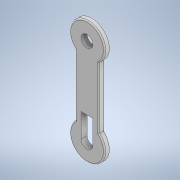
# Autodesk Inventor part: First arm
Saved by Autodesk Inventor 2022 (Build 260153000, 153)
## iProperties
Created: 2022-01-28
Part Number: First arm
Material: Generic
Document SubType Name: Modeling
Designer: Alexa
Density: 1 g/cm^3
Appearance: Default
Author: Alexa
Autodesk Inventor part; units mm, degrees
ref_plane "YZ Plane" through (0, 0, 0) normal (1, 0, 0) x (0, 1, 0)
ref_plane "XZ Plane" through (0, 0, 0) normal (0, 1, 0) x (-1, 0, 0)
ref_plane "XY Plane" through (0, 0, 0) normal (0, 0, 1) x (1, 0, 0)
sketch "Sketch1" plane through (0, 0, 0) normal (0, 0, 1) x (1, 0, 0)
  line L0 (0, 0) -> (20, 0)
  line L1 (20, 0) -> (20, 41)
  line L2 (20, 41) -> (0, 41)
  line L3 (0, 41) -> (0, 0)
  circle A0 centre (10, 0) radius 30
  circle A1 centre (10, 0) radius 10
  line L4 (10, 0) -> (30, 0)
  line L5 (30, 0) -> (30, 150)
  line L6 (30, 150) -> (10, 150)
  line L7 (10, 150) -> (10, 0)
  line L8 (10, 0) -> (-10, 0)
  line L9 (-10, 0) -> (-10, 150)
  line L10 (-10, 150) -> (10, 150)
  line L11 (10, 150) -> (10, 0)
  circle A2 centre (10, 150) radius 30
  circle A3 centre (10, 150) radius 10
  point P0 (30, 22.3607)
  point P1 (30, 127.6393)
  point P2 (-10, 127.6393)
  point P3 (-10, 22.3607)
  dimension "d0" = 20
  dimension "d1" = 41
  dimension "d2" = 60
  dimension "d3" = 20
  dimension "d4" = 150
  dimension "d5" = 20
  dimension "d6" = 150
  dimension "d7" = 60
  dimension "d8" = 20
  constraints: 24 end point, 6 parallel, 3 centre point, 3 coincident, 3 horizontal, 3 perpendicular, 1 horizontal alignment, 1 midpoint, 2 other
  measures "d0" distance of L2.end L1.end
  measures "d1" distance of L1.end L0.end
  measures "d2" diameter of A0
  measures "d3" distance of L6.end L5.end
  measures "d4" distance of L5.end L4.end
  measures "d5" distance of L9.end L10.end
  measures "d6" distance of L8.end L9.end
  measures "d7" diameter of A2
  measures "d8" diameter of A3
extrude "Extrusion1" add sketch "Sketch1" along normal blind 10 contours L8 L9 A0 L3 | L3 A0 L7 A1 | A1 L4 L5 A0 L9 L8 | A0 L9 A2 L7 L2 L3 | L3 L2 L7 A0 | A1 L7 A0 L1 | L1 A0 L5 L4 | L7 L2 L1 A0 | L1 L2 L7 A2 L5 A0 | A2 L5 L6 A3 L10 L9 | L9 L10 A3 L7 A2 | L7 A3 L6 L5 A2
fillet "Fillet1" radius 2 8 edges at (10, 180, 10) (-10, 75, 10) (10, -30, 10) (10, -30, 0) (-10, 75, 0) (10, 180, 0) (30, 75, 0) (30, 75, 10)
sketch "Sketch2" plane through (0, 0, 10) normal (0, 0, 1) x (1, 0, 0)
  line L0 (0, 0) -> (20, 0)
  line L1 (20, 0) -> (20, 40.5)
  line L2 (20, 40.5) -> (0, 40.5)
  line L3 (0, 40.5) -> (0, 0)
  dimension "d12" = 20
  dimension "d13" = 40.5
  constraints: 8 end point, 2 parallel, 1 horizontal, 1 perpendicular
  measures "d12" distance of L2.end L1.end
  measures "d13" distance of L1.end L0.end
extrude "Extrusion2" cut sketch "Sketch2" against normal blind 10.6375
body "Solid1"
